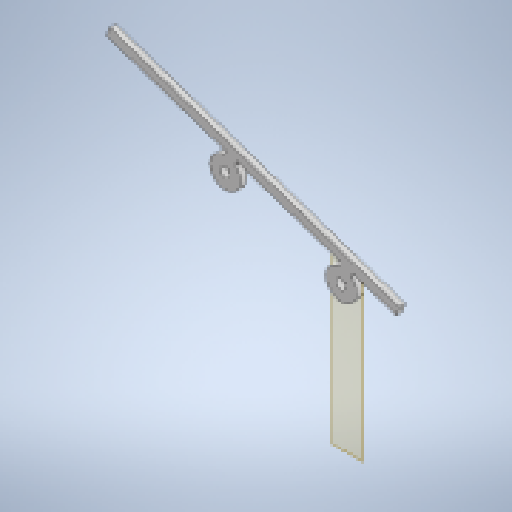
# Autodesk Inventor part: leaf-lid
Saved by Autodesk Inventor 2024.1 (Build 281209000, 209)
## iProperties
Created: 2025-06-11
Part Number: leaf-lid
Material: Generic
Document SubType Name: Modeling
Designer: iwheard
Density: 1 g/cm^3
Appearance: Default
Author: iwheard
Autodesk Inventor part; units mm, degrees
ref_plane "YZ Plane" through (0, 0, 0) normal (1, 0, 0) x (0, 1, 0)
ref_plane "XZ Plane" through (0, 0, 0) normal (0, 1, 0) x (-1, 0, 0)
ref_plane "XY Plane" through (0, 0, 0) normal (0, 0, 1) x (1, 0, 0)
ref_plane "Work Plane1" through (0, 0, 0) normal (0, 0, 1) x (1, 0, 0)
sketch "Sketch1" plane through (0, 0, 0) normal (0, 0, 1) x (1, 0, 0)
  circle A0 centre (0, 28) radius 1.6 projected
  arc A1 (3.5119, -2.971) -> (3.88, 2.471) centre (0, 0) ccw projected
  arc A2 (4.2226, 26.7696) -> (3.88, 2.471) centre (48.0455, 14) ccw projected
  arc A3 (4.2226, 26.7696) -> (-4.2226, 26.7696) centre (0, 28) ccw projected
  arc A4 (-3.88, 2.471) -> (-4.2226, 26.7696) centre (-48.0455, 14) ccw projected
  arc A5 (-3.88, 2.471) -> (-3.5119, -2.971) centre (0, 0) ccw projected
  arc A6 (-3.9828, -12.5413) -> (-3.5119, -2.971) centre (-19.1125, -7) ccw projected
  arc A7 (-3.9828, -12.5413) -> (3.9828, -12.5413) centre (0, -14) ccw projected
  arc A8 (3.5119, -2.971) -> (3.9828, -12.5413) centre (19.1125, -7) ccw projected
  circle A9 centre (0, 0) radius 1.6 projected
  circle A10 centre (0, 21) radius 1.6 projected
  circle A11 centre (0, 28) radius 1.6 projected
  circle A12 centre (0, 14) radius 1.6 projected
  circle A13 centre (0, 7) radius 1.6 projected
  circle A14 centre (0, -7) radius 1.6 projected
  circle A15 centre (0, -14) radius 1.6 projected
  circle A16 centre (0, 28) radius 5
  line L0 (18, 28.1562) -> (18.9553, 31)
  line L1 (18.9553, 31) -> (-75.839, 62.8438)
  line L2 (-75.839, 62.8438) -> (-76.7944, 60)
  line L3 (-76.7944, 60) -> (18, 28.1562)
  line L4 (3.7683, 32.937) -> (-0.0235, 34.2107)
  line L5 (-0.0235, 34.2107) -> (-0.4366, 32.9809)
  line L6 (-0.4366, 32.9809) -> (3.3552, 31.7071)
  line L7 (3.3552, 31.7071) -> (3.7683, 32.937)
  line L8 (9.4559, 31.0263) -> (9.0428, 29.7965)
  circle A17 centre (9.4794, 24.8156) radius 5
  line L9 (9.0428, 29.7965) -> (12.8346, 28.5228)
  line L10 (12.8346, 28.5228) -> (13.2477, 29.7526)
  line L11 (-9.5029, 37.3951) -> (-9.9161, 36.1653)
  circle A18 centre (-9.4794, 31.1844) radius 5
  line L12 (-9.9161, 36.1653) -> (-6.1243, 34.8915)
  line L13 (-6.1243, 34.8915) -> (-5.7112, 36.1213)
  line L14 (-0.0235, 34.2107) -> (-0.4366, 32.9809)
  circle A19 centre (0, 28) radius 5
  line L15 (-0.4366, 32.9809) -> (3.3552, 31.7071)
  line L16 (3.3552, 31.7071) -> (3.7683, 32.937)
  line L17 (-18.9824, 40.5795) -> (-19.3955, 39.3497)
  circle A20 centre (-18.9589, 34.3688) radius 5
  line L18 (-19.3955, 39.3497) -> (-15.6037, 38.0759)
  line L19 (-15.6037, 38.0759) -> (-15.1906, 39.3057)
  line L20 (-9.5029, 37.3951) -> (-9.9161, 36.1653)
  circle A21 centre (-9.4794, 31.1844) radius 5
  line L21 (-9.9161, 36.1653) -> (-6.1243, 34.8915)
  line L22 (-6.1243, 34.8915) -> (-5.7112, 36.1213)
  line L23 (-28.4618, 43.7639) -> (-28.8749, 42.534)
  circle A22 centre (-28.4383, 37.5531) radius 5
  line L24 (-28.8749, 42.534) -> (-25.0832, 41.2603)
  line L25 (-25.0832, 41.2603) -> (-24.67, 42.4901)
  line L26 (-18.9824, 40.5795) -> (-19.3955, 39.3497)
  circle A23 centre (-18.9589, 34.3688) radius 5
  line L27 (-19.3955, 39.3497) -> (-15.6037, 38.0759)
  line L28 (-15.6037, 38.0759) -> (-15.1906, 39.3057)
  line L29 (-37.9412, 46.9483) -> (-38.3544, 45.7184)
  circle A24 centre (-37.9177, 40.7375) radius 5
  line L30 (-38.3544, 45.7184) -> (-34.5626, 44.4447)
  line L31 (-34.5626, 44.4447) -> (-34.1495, 45.6745)
  line L32 (-28.4618, 43.7639) -> (-28.8749, 42.534)
  circle A25 centre (-28.4383, 37.5531) radius 5
  line L33 (-28.8749, 42.534) -> (-25.0832, 41.2603)
  line L34 (-25.0832, 41.2603) -> (-24.67, 42.4901)
  line L35 (-47.4207, 50.1326) -> (-47.8338, 48.9028)
  circle A26 centre (-47.3972, 43.9219) radius 5
  line L36 (-47.8338, 48.9028) -> (-44.042, 47.6291)
  line L37 (-44.042, 47.6291) -> (-43.6289, 48.8589)
  line L38 (-37.9412, 46.9483) -> (-38.3544, 45.7184)
  circle A27 centre (-37.9177, 40.7375) radius 5
  line L39 (-38.3544, 45.7184) -> (-34.5626, 44.4447)
  line L40 (-34.5626, 44.4447) -> (-34.1495, 45.6745)
  line L41 (-56.9001, 53.317) -> (-57.3132, 52.0872)
  circle A28 centre (-56.8766, 47.1063) radius 5
  line L42 (-57.3132, 52.0872) -> (-53.5215, 50.8134)
  line L43 (-53.5215, 50.8134) -> (-53.1083, 52.0433)
  line L44 (-47.4207, 50.1326) -> (-47.8338, 48.9028)
  circle A29 centre (-47.3972, 43.9219) radius 5
  line L45 (-47.8338, 48.9028) -> (-44.042, 47.6291)
  line L46 (-44.042, 47.6291) -> (-43.6289, 48.8589)
  line L47 (-66.3795, 56.5014) -> (-66.7927, 55.2716)
  circle A30 centre (-66.3561, 50.2907) radius 5
  line L48 (-66.7927, 55.2716) -> (-63.0009, 53.9978)
  line L49 (-63.0009, 53.9978) -> (-62.5878, 55.2276)
  line L50 (-56.9001, 53.317) -> (-57.3132, 52.0872)
  circle A31 centre (-56.8766, 47.1063) radius 5
  line L51 (-57.3132, 52.0872) -> (-53.5215, 50.8134)
  line L52 (-53.5215, 50.8134) -> (-53.1083, 52.0433)
  line L53 (-75.859, 59.6858) -> (-76.2721, 58.456)
  circle A32 centre (-75.8355, 53.4751) radius 5
  line L54 (-76.2721, 58.456) -> (-72.4803, 57.1822)
  line L55 (-72.4803, 57.1822) -> (-72.0672, 58.412)
  line L56 (-66.3795, 56.5014) -> (-66.7927, 55.2716)
  circle A33 centre (-66.3561, 50.2907) radius 5
  line L57 (-66.7927, 55.2716) -> (-63.0009, 53.9978)
  line L58 (-63.0009, 53.9978) -> (-62.5878, 55.2276)
  circle A34 centre (0, 28) radius 1.6
  circle A35 centre (-9.4794, 31.1844) radius 1.6
  circle A36 centre (-18.9589, 34.3688) radius 1.6
  circle A37 centre (-28.4383, 37.5531) radius 1.6
  circle A38 centre (-37.9177, 40.7375) radius 1.6
  circle A39 centre (-47.3972, 43.9219) radius 1.6
  circle A40 centre (-56.8766, 47.1063) radius 1.6
  circle A41 centre (-66.3561, 50.2907) radius 1.6
  circle A42 centre (-75.8355, 53.4751) radius 1.6
  circle A43 centre (9.4794, 24.8156) radius 1.6
  circle A44 centre (0, 28) radius 1.6
  circle A45 centre (-9.4794, 31.1844) radius 1.6
  circle A46 centre (-18.9589, 34.3688) radius 1.6
  circle A47 centre (-28.4383, 37.5531) radius 1.6
  circle A48 centre (-37.9177, 40.7375) radius 1.6
  circle A49 centre (-47.3972, 43.9219) radius 1.6
  circle A50 centre (-56.8766, 47.1063) radius 1.6
  circle A51 centre (-66.3561, 50.2907) radius 1.6
  dimension "d0" = 10
  dimension "d1" = 18
  dimension "d2" = 3
  dimension "d3" = 3
  dimension "d4" = 100
  dimension "d5" = 32
  dimension "d6" = 4
  dimension "d11" = 10
  dimension "d14" = 10
  dimension "d19" = 10
  dimension "d22" = 10
  constraints: 118 end point, 36 centre point, 36 point on circle, 4 parallel, 2 coincident, 2 perpendicular, 2 point on line, 1 concentric, 191 other
  measures "d0" diameter of A16
  measures "d1" horizontal distance of L0.start A0.centre
  measures "d2" distance between parallel lines of L1 L3
  measures "d3" vertical distance of L0.end A0.centre
  measures "d4" distance between parallel lines of L2 L0
  measures "d5" vertical distance of L2.end A0.centre
  measures "d6" distance between parallel lines of L5 L7
  measures "d11" distance of L4.end L8.start
  measures "d14" distance of L4.end L11.start
  measures "d19" distance of A34.centre A35.centre
  measures "d22" distance of A34.centre A43.centre
extrude "Extrusion1" add sketch "Sketch1" along normal blind 2 contours A16 A4 A3 A2 | A2 A3 A4 A16 L6 | L5 L3 L7 A16 | A16 L6 | L3 L2 L1 L0 | A24 L30 | L29 L3 L31 A24 | A24 L30
body "Solid1"
